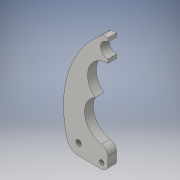
# Autodesk Inventor part: GripperFingersExtended
Saved by Autodesk Inventor 2016 (Build 200138000, 138)
## iProperties
Created: 2016-08-23
Part Number: GripperFingersExtended
Material: Generic
Document SubType Name: Modeling
Designer: lachesis
Density: 1 g/cm^3
Appearance: Default
Author: lachesis
Autodesk Inventor part; units mm, degrees
ref_plane "YZ Plane" through (0, 0, 0) normal (1, 0, 0) x (0, 1, 0)
ref_plane "XZ Plane" through (0, 0, 0) normal (0, 1, 0) x (-1, 0, 0)
ref_plane "XY Plane" through (0, 0, 0) normal (0, 0, 1) x (1, 0, 0)
sketch "Sketch2" plane through (0, 0, 0) normal (0, 0, 1) x (1, 0, 0)
  line L0 (13.0302, 41.5925) -> (13.0302, -41.5925)
  line L1 (13.0302, -41.5925) -> (-13.0302, -41.5925)
  arc A0 (13.0302, 41.5925) -> (-13.0302, -41.5925) centre (53.0449, -16.618) ccw
  point P0 (0, 0)
  point P1 (13.0302, 0)
  point P2 (0, -41.5925)
  dimension "d6" = 26.0604
  dimension "d32" = 70.6374
  dimension "d33" = 83.185
  constraints: 4 end point, 2 midpoint, 2 point on circle, 1 centre point, 1 horizontal, 1 horizontal alignment, 1 vertical, 1 vertical alignment
  measures "d6" distance of L0.end L1.end
  measures "d32" radius of A0
  measures "d33" distance of L0.end L0.start
extrude "Extrusion1" add sketch "Sketch2" along normal blind 6
fillet "Fillet2" radius 7.8 1 edges at (-13.0302, -41.5925, 3)
fillet "Fillet3" radius 4.33 1 edges at (13.0302, -41.5925, 3)
sketch "Sketch6" plane through (0, 0, 6) normal (0, 0, 1) x (1, 0, 0)
  line L0 (13.0302, -37.2625) -> (13.0302, 41.5925) projected
  arc A0 (8.7002, -41.5925) -> (13.0302, -37.2625) centre (8.7002, -37.2625) ccw projected
  line L1 (13.0302, -37.2625) -> (13.0302, 41.5925) projected
  arc A1 (13.0302, 41.5925) -> (-14.9029, -35.9244) centre (53.0449, -16.618) ccw projected
  arc A2 (-14.9029, -35.9244) -> (-7.3999, -41.5925) centre (-7.3999, -33.7925) ccw projected
  line L2 (-7.3999, -41.5925) -> (8.7002, -41.5925) projected
  arc A3 (4.2419, -1.0136) -> (13.0302, -26.6511) centre (10.6426, -13.1445) ccw
  line L3 (13.0302, 0.3621) -> (13.0302, -26.6511)
  arc A4 (13.0302, 23.8159) -> (4.2419, -1.0136) centre (13.0302, 9.8459) ccw
  line L4 (13.0302, 0.3621) -> (13.0302, -4.1241)
  line L5 (13.0302, 0.3621) -> (13.0302, 23.8159)
  point P0 (0, 0)
  dimension "d37" = 2.3876
  dimension "d38" = 13.716
  dimension "d39" = 14.732
  dimension "d41" = 50.8
  dimension "d42" = 13.97
  constraints: 6 end point, 5 point on circle, 4 point on line, 2 centre point, 1 collinear
  measures "d37" distance from line of A3.centre L0
  measures "d38" radius of A3
  measures "d39" distance edge to line of A3 L2
  measures "d42" radius of A4
extrude "Extrusion4" cut sketch "Sketch6" against normal through all contours A3 A4 L0
sketch "Sketch7" plane through (0, 0, 6) normal (0, 0, 1) x (1, 0, 0)
  arc A0 (13.0302, 23.8159) -> (4.2419, -1.0136) centre (13.0302, 9.8459) ccw projected
  line L0 (13.0302, 23.8159) -> (13.0302, 41.5925) projected
  arc A1 (13.0302, 41.5925) -> (-14.9029, -35.9244) centre (53.0449, -16.618) ccw projected
  arc A2 (-14.9029, -35.9244) -> (-7.3999, -41.5925) centre (-7.3999, -33.7925) ccw projected
  line L1 (-7.3999, -41.5925) -> (8.7002, -41.5925) projected
  arc A3 (8.7002, -41.5925) -> (13.0302, -37.2625) centre (8.7002, -37.2625) ccw projected
  line L2 (13.0302, -37.2625) -> (13.0302, -26.6511) projected
  arc A4 (4.2419, -1.0136) -> (13.0302, -26.6511) centre (10.6426, -13.1445) ccw projected
  line L3 (13.0302, 23.8159) -> (13.0302, 41.5925) projected
  line L4 (13.0302, 23.8159) -> (17.2669, 23.8159) construction
  arc A5 (13.0302, 36.5159) -> (13.0302, 26.3559) centre (13.0302, 31.4359) ccw
  line L5 (13.0302, 36.5159) -> (13.0302, 26.3559)
  point P0 (0, 0)
  dimension "d46" = 10.16
  dimension "d47" = 2.54
  constraints: 4 end point, 3 point on line, 2 point on circle, 1 centre point, 1 horizontal
  measures "d46" diameter of A5
  measures "d47" distance edge to line of A5 L4
extrude "Extrusion5" cut sketch "Sketch7" against normal through all contours A5 L0
sketch "Sketch8" plane through (0, 0, 6) normal (0, 0, 1) x (1, 0, 0)
  arc A0 (13.0302, 36.5159) -> (13.0302, 26.3559) centre (13.0302, 31.4359) ccw projected
  line L0 (13.0302, 36.5159) -> (13.0302, 41.5925) projected
  arc A1 (13.0302, 41.5925) -> (-14.9029, -35.9244) centre (53.0449, -16.618) ccw projected
  arc A2 (-14.9029, -35.9244) -> (-7.3999, -41.5925) centre (-7.3999, -33.7925) ccw projected
  line L1 (-7.3999, -41.5925) -> (8.7002, -41.5925) projected
  arc A3 (8.7002, -41.5925) -> (13.0302, -37.2625) centre (8.7002, -37.2625) ccw projected
  line L2 (13.0302, -37.2625) -> (13.0302, -26.6511) projected
  arc A4 (4.2419, -1.0136) -> (13.0302, -26.6511) centre (10.6426, -13.1445) ccw projected
  arc A5 (13.0302, 23.8159) -> (4.2419, -1.0136) centre (13.0302, 9.8459) ccw projected
  line L3 (13.0302, 23.8159) -> (13.0302, 26.3559) projected
  line L4 (13.0302, 39.0559) -> (9.5701, 39.0559)
  arc A6 (13.0302, 41.5925) -> (-14.9029, -35.9244) centre (53.0449, -16.618) ccw projected
  line L5 (13.0302, 36.5159) -> (13.0302, 41.5925) projected
  point P0 (0, 0)
  dimension "d50" = 2.54
  constraints: 2 end point, 2 point on circle, 1 perpendicular, 1 point on line
  measures "d50" distance from line of L0.start L4
extrude "Extrusion6" cut sketch "Sketch8" against normal through all contours L4 A1 L0
fillet "Fillet4" radius 5.051 1 edges at (13.0302, -26.6511, 3)
sketch "Sketch9" plane through (0, 0, 6) normal (0, 0, 1) x (1, 0, 0)
  arc A0 (13.0302, -31.7215) -> (8.696, -26.7217) centre (7.9792, -31.7215) ccw projected
  arc A1 (4.2419, -1.0136) -> (8.696, -26.7217) centre (10.6426, -13.1445) ccw projected
  arc A2 (13.0302, 23.8159) -> (4.2419, -1.0136) centre (13.0302, 9.8459) ccw projected
  line L0 (13.0302, 23.8159) -> (13.0302, 26.3559) projected
  arc A3 (13.0302, 36.5159) -> (13.0302, 26.3559) centre (13.0302, 31.4359) ccw projected
  arc A4 (9.5701, 39.0559) -> (-14.9029, -35.9244) centre (53.0449, -16.618) ccw projected
  arc A5 (-14.9029, -35.9244) -> (-7.3999, -41.5925) centre (-7.3999, -33.7925) ccw projected
  line L1 (-7.3999, -41.5925) -> (8.7002, -41.5925) projected
  arc A6 (8.7002, -41.5925) -> (13.0302, -37.2625) centre (8.7002, -37.2625) ccw projected
  line L2 (13.0302, -37.2625) -> (13.0302, -31.7215) projected
  circle A7 centre (8.9027, -37.465) radius 1.5875
  circle A8 centre (-7.0993, -33.8074) radius 1.8415
  line L3 (13.0302, 36.5159) -> (13.0302, 39.0559) projected
  line L4 (13.0302, 39.0559) -> (9.5701, 39.0559) projected
  point P0 (0, 0)
  dimension "d54" = 2.54
  dimension "d55" = 2.54
  dimension "d56" = 3.175
  dimension "d57" = 5.9436
  dimension "d58" = 16.002
  dimension "d59" = 3.683
  constraints: 2 centre point
  measures "d54" distance edge to line of A7 L1
  measures "d55" distance edge to line of A7 L2
  measures "d56" diameter of A7
  measures "d57" distance edge to line of A8 L1
  measures "d58" horizontal distance of A7.centre A8.centre
  measures "d59" diameter of A8
extrude "Extrusion7" cut sketch "Sketch9" against normal through all contours A7 | A8
body "Solid1"
